Autodesk Inventor part; units mm, degrees
(part 4 of 4)
  circle A1496 centre (8.17, -62.94) radius 0.625
  circle A1497 centre (10.71, -62.94) radius 0.625
  circle A1498 centre (13.25, -62.94) radius 0.625
  circle A1499 centre (15.79, -62.94) radius 0.625
  circle A1500 centre (18.33, -62.94) radius 0.625
  circle A1501 centre (20.87, -62.94) radius 0.625
  circle A1502 centre (23.41, -62.94) radius 0.625
  circle A1503 centre (25.95, -62.94) radius 0.625
  circle A1504 centre (28.49, -62.94) radius 0.625
  circle A1505 centre (31.03, -62.94) radius 0.625
  circle A1506 centre (33.57, -62.94) radius 0.625
  circle A1507 centre (36.11, -62.94) radius 0.625
  circle A1508 centre (38.65, -62.94) radius 0.625
  circle A1509 centre (41.19, -62.94) radius 0.625
  circle A1510 centre (43.73, -62.94) radius 0.625
  circle A1511 centre (46.27, -62.94) radius 0.625
  circle A1512 centre (48.81, -62.94) radius 0.625
  circle A1513 centre (51.35, -62.94) radius 0.625
  circle A1514 centre (53.89, -62.94) radius 0.625
  circle A1515 centre (56.43, -62.94) radius 0.625
  circle A1516 centre (58.97, -62.94) radius 0.625
  circle A1517 centre (61.51, -62.94) radius 0.625
  circle A1518 centre (64.05, -62.94) radius 0.625
  circle A1519 centre (66.59, -62.94) radius 0.625
  circle A1520 centre (69.13, -62.94) radius 0.625
  circle A1521 centre (71.67, -62.94) radius 0.625
  circle A1522 centre (74.21, -62.94) radius 0.625
  circle A1523 centre (76.75, -62.94) radius 0.625
  circle A1524 centre (79.29, -62.94) radius 0.625
  circle A1525 centre (81.83, -62.94) radius 0.625
  circle A1526 centre (8.17, -65.48) radius 0.625
  circle A1527 centre (10.71, -65.48) radius 0.625
  circle A1528 centre (13.25, -65.48) radius 0.625
  circle A1529 centre (15.79, -65.48) radius 0.625
  circle A1530 centre (18.33, -65.48) radius 0.625
  circle A1531 centre (20.87, -65.48) radius 0.625
  circle A1532 centre (23.41, -65.48) radius 0.625
  circle A1533 centre (25.95, -65.48) radius 0.625
  circle A1534 centre (28.49, -65.48) radius 0.625
  circle A1535 centre (31.03, -65.48) radius 0.625
  circle A1536 centre (33.57, -65.48) radius 0.625
  circle A1537 centre (36.11, -65.48) radius 0.625
  circle A1538 centre (38.65, -65.48) radius 0.625
  circle A1539 centre (41.19, -65.48) radius 0.625
  circle A1540 centre (43.73, -65.48) radius 0.625
  circle A1541 centre (46.27, -65.48) radius 0.625
  circle A1542 centre (48.81, -65.48) radius 0.625
  circle A1543 centre (51.35, -65.48) radius 0.625
  circle A1544 centre (53.89, -65.48) radius 0.625
  circle A1545 centre (56.43, -65.48) radius 0.625
  circle A1546 centre (58.97, -65.48) radius 0.625
  circle A1547 centre (61.51, -65.48) radius 0.625
  circle A1548 centre (64.05, -65.48) radius 0.625
  circle A1549 centre (66.59, -65.48) radius 0.625
  circle A1550 centre (69.13, -65.48) radius 0.625
  circle A1551 centre (71.67, -65.48) radius 0.625
  circle A1552 centre (74.21, -65.48) radius 0.625
  circle A1553 centre (76.75, -65.48) radius 0.625
  circle A1554 centre (79.29, -65.48) radius 0.625
  circle A1555 centre (81.83, -65.48) radius 0.625
  dimension "d45" = 1.25
  dimension "d48" = 2.54
  dimension "d51" = 2.54
  constraints: 750 centre point, 750 coincident, 1 horizontal, 1 vertical, 2247 other
  measures "d45" diameter of A806
  measures "d48" distance of A806.centre A807.centre
  measures "d51" distance of A806.centre A836.centre
extrude "PCB_Through_Holes" cut sketch "Sketch6" against normal through all
sketch "Sketch7" plane through (0, 1, 0) normal (0, 1, 0) x (1, 0, 0)
  point P0 (0, 0)
body "Solid1"
